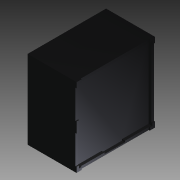
# Autodesk Inventor part: UB216SKG0035-NR
Saved by Autodesk Inventor 2015 SP1 (Build 190203100, 203)
## iProperties
Category: Electrical
Company: Autodesk Inc.
Created: 2014-12-16
Part Number: UB216SKG0035-NR
Catalog Web Link: http://www.nkkswitches.com/
Description: PC and Snap-in Mount Non-Illuminated Pushbuttons_ni_body-Non-Illuminated Pushbuttons - Series UB2
Vendor: NKK Switches
Document SubType Name: Modeling
Designer: Autodesk Inc.
Manufacturer: NKKSWITCHES
Mass: 2.15667 g
Surface Area: 10.8004 cm^2
Volume: 2.15667 cm^3
Density: 1 g/cm^3
Material: Generic
Appearance: PSOLRGB-192-192-192
Title: UB21SK035C-5Dni_body
Author: Autodesk Inc.
Comments: Non-Illuminated Pushbuttons - Series UB2
Autodesk Inventor part; units mm, degrees
sketch "Sketch_2" plane through (1.016, 0, 0) normal (1, 0, 0) x (0, 0, -1)
  line L0 (-7.62, -7.62) -> (7.62, -7.62)
  line L1 (7.62, -7.62) -> (7.62, 7.62)
  line L2 (7.62, 7.62) -> (-7.62, 7.62)
  line L3 (-7.62, 7.62) -> (-7.62, -7.62)
  constraints: 8 end point
extrude "Extrusion1" add sketch "Sketch_2" against normal blind 10.0076
sketch "Sketch_1" plane through (1.016, 0, 0) normal (1, 0, 0) x (0, 0, -1)
  line L0 (-7.112, -7.112) -> (-1.9812, -7.112)
  line L1 (-1.9812, -7.112) -> (-1.9812, -7.366)
  line L2 (-1.9812, -7.366) -> (1.9812, -7.366)
  line L3 (1.9812, -7.366) -> (1.9812, -7.112)
  line L4 (1.9812, -7.112) -> (7.112, -7.112)
  line L5 (7.112, -7.112) -> (7.112, 7.112)
  line L6 (7.112, 7.112) -> (-7.112, 7.112)
  line L7 (-7.112, 7.112) -> (-7.112, -7.112)
  constraints: 16 end point
extrude "Extrusion2" cut sketch "Sketch_1" against normal blind 0.762
sketch "Sketch_3" plane through (0, 0, 0) normal (0, 0, 1) x (1, 0, 0)
  line L0 (-18.9992, 7.62) -> (-18.9992, -7.62)
  line L1 (-18.9992, -7.62) -> (-8.4836, -7.62)
  line L2 (-8.4836, -7.62) -> (-8.9916, -7.112)
  line L3 (-8.9916, -7.112) -> (-8.9916, 7.112)
  line L4 (-8.9916, 7.112) -> (-8.4836, 7.62)
  line L5 (-8.4836, 7.62) -> (-18.9992, 7.62)
  constraints: 12 end point
extrude "Extrusion3" cut sketch "Sketch_3" along normal mid plane 15.24
sketch "Sketch_4" plane through (0, 0, 0) normal (0, 1, 0) x (-1, 0, 0)
  line L0 (18.9992, -7.62) -> (18.9992, 7.62)
  line L1 (18.9992, 7.62) -> (8.4836, 7.62)
  line L2 (8.4836, 7.62) -> (8.9916, 7.112)
  line L3 (8.9916, 7.112) -> (8.9916, -7.112)
  line L4 (8.9916, -7.112) -> (8.4836, -7.62)
  line L5 (8.4836, -7.62) -> (18.9992, -7.62)
  constraints: 12 end point
extrude "Extrusion4" cut sketch "Sketch_4" along normal mid plane 15.24
sketch "Sketch_5" plane through (0, 7.62, 0) normal (0, 1, 0) x (1, 0, 0)
  line L0 (0.8128, 6.604) -> (0.8128, -6.604)
  line L1 (0.8128, -6.604) -> (1.016, -6.604)
  line L2 (1.016, -6.604) -> (1.016, 6.604)
  line L3 (1.016, 6.604) -> (0.8128, 6.604)
  constraints: 8 end point
extrude "Extrusion5" cut sketch "Sketch_5" against normal blind 15.24
sketch "Sketch_6" plane through (0, 0, -7.62) normal (0, 0, 1) x (1, 0, 0)
  line L0 (0.8128, 6.604) -> (0.8128, -6.604)
  line L1 (0.8128, -6.604) -> (1.016, -6.604)
  line L2 (1.016, -6.604) -> (1.016, 6.604)
  line L3 (1.016, 6.604) -> (0.8128, 6.604)
  constraints: 8 end point
extrude "Extrusion6" cut sketch "Sketch_6" along normal blind 0.508
sketch "Sketch_7" plane through (0, 0, 7.62) normal (0, 0, 1) x (1, 0, 0)
  line L0 (0.8128, 6.604) -> (0.8128, 1.016)
  line L1 (0.8128, 1.016) -> (1.016, 1.016)
  line L2 (1.016, 1.016) -> (1.016, 6.604)
  line L3 (1.016, 6.604) -> (0.8128, 6.604)
  constraints: 8 end point
extrude "Extrusion7" cut sketch "Sketch_7" against normal blind 0.508
sketch "Sketch_8" plane through (0, 0, 7.62) normal (0, 0, 1) x (1, 0, 0)
  line L0 (0.8128, -1.016) -> (0.8128, -6.604)
  line L1 (0.8128, -6.604) -> (1.016, -6.604)
  line L2 (1.016, -6.604) -> (1.016, -1.016)
  line L3 (1.016, -1.016) -> (0.8128, -1.016)
  constraints: 8 end point
extrude "Extrusion8" cut sketch "Sketch_8" against normal blind 0.508
ref_plane "body_to_dummy_sk_XY" through (-11.4046, 0, 0) normal (-1, 0, 0) x (0, 0, -1)
ref_plane "body_to_dummy_sk_YZ" through (-11.4046, 0, 0) normal (0, 0, -1) x (0, -1, 0)
ref_plane "body_to_dummy_sk_ZX" through (-11.4046, 0, 0) normal (0, -1, 0) x (-1, 0, 0)
ref_plane "body_to_pole_XY" through (-0.508, 0, 0) normal (-1, 0, 0) x (0, 0, -1)
ref_plane "body_to_pole_YZ" through (-0.508, 0, 0) normal (0, 0, -1) x (0, -1, 0)
ref_plane "body_to_pole_ZX" through (-0.508, 0, 0) normal (0, -1, 0) x (-1, 0, 0)
body "Solid1"
